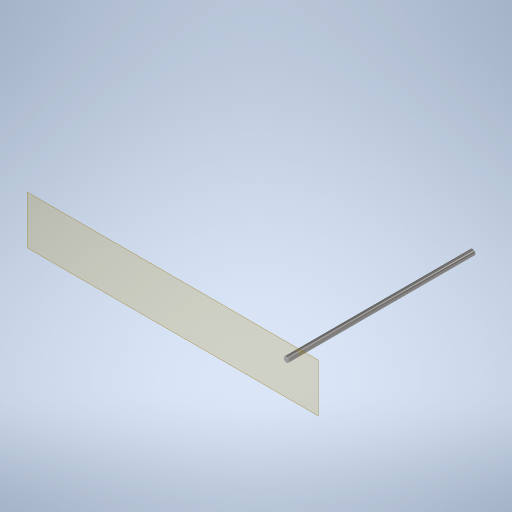
# Autodesk Inventor part: pin
Saved by Autodesk Inventor 2023 (Build 270158030, 158C)
## iProperties
Created: 2023-04-28
Part Number: pin
Material: Generic
Document SubType Name: Modeling
Designer: Imogen Heard
Density: 1 g/cm^3
Appearance: Default
Author: Imogen Heard
Autodesk Inventor part; units mm, degrees
ref_plane "YZ Plane" through (0, 0, 0) normal (1, 0, 0) x (0, 1, 0)
ref_plane "XZ Plane" through (0, 0, 0) normal (0, 1, 0) x (-1, 0, 0)
ref_plane "XY Plane" through (0, 0, 0) normal (0, 0, 1) x (1, 0, 0)
ref_plane "Work Plane1" through (0, 0, 0) normal (0, 0, 1) x (1, 0, 0)
sketch "Sketch1" plane through (0, 0, 0) normal (0, 0, 1) x (1, 0, 0)
  arc A0 (77.7774, 1.7905) -> (78.5846, 1.4138) centre (77.9, 1) ccw projected
  circle A1 centre (77.9, 1) radius 0.8
  point P0 (0, 0)
  point P1 (78.5846, 1.4138)
  dimension "d0" = 1.6
  constraints: 1 centre point, 1 concentric
  measures "d0" diameter of A1
extrude "Extrusion1" add sketch "Sketch1" along normal blind 3 and the other way blind 53
body "Solid1"
